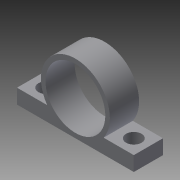
# Autodesk Inventor part: Pillow block for arm bearing
Saved by Autodesk Inventor 2013 (Build 170138000, 138)
## iProperties
Created: 2013-02-02
Part Number: Pillow block for arm bearing
Material: Aluminum 6061
Document SubType Name: Sheet Metal
Designer: aslane
Density: 1 g/cm^3
Sheet Metal Rule: Default
Author: aslane
Autodesk Inventor part; units mm, degrees
ref_plane "YZ Plane" through (0, 0, 0) normal (1, 0, 0) x (0, 1, 0)
ref_plane "XZ Plane" through (0, 0, 0) normal (0, 1, 0) x (-1, 0, 0)
ref_plane "XY Plane" through (0, 0, 0) normal (0, 0, 1) x (1, 0, 0)
sketch "Sketch1" plane through (0, 0, 0) normal (0, 0, 1) x (1, 0, 0)
  line L0 (0, 0) -> (50.8, 0)
  arc A0 (37.6547, 6.35) -> (13.1453, 6.35) centre (25.4, 15) ccw
  circle A1 centre (25.4, 15) radius 13
  line L1 (0, 0) -> (0, 6.35)
  line L2 (0, 6.35) -> (13.1453, 6.35)
  line L3 (50.8, 0) -> (50.8, 6.35)
  line L4 (50.8, 6.35) -> (37.6547, 6.35)
  dimension "d0" = 50.8
  dimension "d1" = 30
  dimension "d2" = 26
  dimension "d3" = 6.35
  dimension "d4" = 6.35
  dimension "d5" = 25.4
  measures "d0" distance of L0.start L0.end
  measures "d1" diameter of A0
  measures "d2" diameter of A1
  measures "d3" distance of L0.start L1.end
  measures "d4" distance of L0.end L3.end
  measures "d5" distance from line of L3 A1.centre
extrude "Plate1" add sketch "Sketch1" along normal blind 12.7
sketch "Sketch2" plane through (37.6547, 6.35, 0) normal (0, 1, 0) x (1, 0, 0)
  line L0 (0, -12.7) -> (13.1453, -12.7) projected
  line L1 (13.1453, 0) -> (13.1453, -12.7) projected
  circle A0 centre (6.7953, -6.35) radius 3.3782
  circle A1 centre (-31.3047, -6.35) radius 3.3782
  line L2 (-37.6547, 0) -> (-37.6547, -12.7) projected
  line L3 (-24.5094, 0) -> (-37.6547, 0) projected
  dimension "d7" = 6.7564
  dimension "d8" = 6.7564
  dimension "d9" = 6.35
  dimension "d10" = 6.35
  dimension "d12" = 6.35
  dimension "d13" = 6.35
  constraints: 2 centre point
  measures "d7" diameter of A0
  measures "d8" diameter of A1
  measures "d9" distance from line of L1 A0.centre
  measures "d10" distance from line of L0 A0.centre
  measures "d12" distance from line of L2 A1.centre
  measures "d13" distance from line of L3 A1.centre
extrude "Cut1" cut sketch "Sketch2" against normal blind 12.7
equation "\"d14\" = Thickness"
equation "\"BendRadius\" = Thickness"
equation "\"BendReliefWidth\" = Thickness"
equation "\"BendReliefDepth\" = 0.5 * Thickness"
equation "\"CornerReliefSize\" = 4 * Thickness"
equation "\"MinimumRemnant\" = 2 * Thickness"
equation "\"TransitionRadius\" = BendRadius"
equation "\"JacobiRadiusSize\" = BendRadius"
equation "\"GapSize\" = Thickness"
equation "\"d6\" = BendRadius"
equation "\"Thickness\" = 12.7"
body "Solid1"
